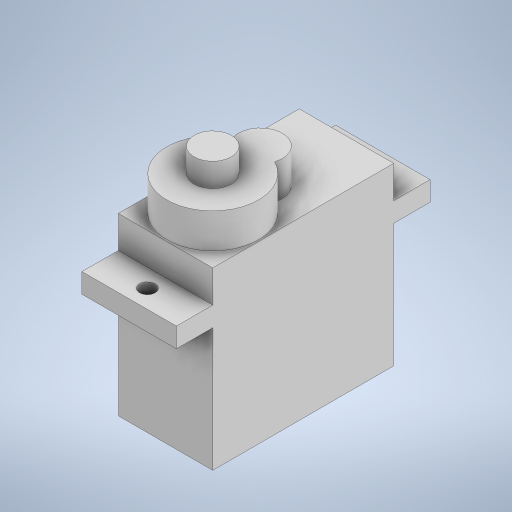
# Autodesk Inventor part: Servo Motor
Saved by Autodesk Inventor 2023 (Build 270158000, 158)
## iProperties
Created: 2023-03-09
Part Number: Servo Motor
Material: Generic
Document SubType Name: Modeling
Designer: 1roweste
Density: 1 g/cm^3
Appearance: Default
Author: 1roweste
Autodesk Inventor part; units mm, degrees
ref_plane "YZ Plane" through (0, 0, 0) normal (1, 0, 0) x (0, 1, 0)
sketch "Sketch1" plane through (0, 0, 0) normal (0, 1, 0) x (-1, 0, 0)
  line L0 (-6, 11.5) -> (6, 11.5)
  line L1 (6, 11.5) -> (6, -11.5)
  line L2 (6, -11.5) -> (-6, -11.5)
  line L3 (-6, -11.5) -> (-6, 11.5)
  point P0 (0, 0)
  point P1 (6, 0)
  point P2 (0, -11.5)
  dimension "d0" = 12
  dimension "d1" = 23
  dimension "d2" = 0
  dimension "d3" = 0
  constraints: 8 end point, 2 midpoint, 2 parallel, 1 horizontal, 1 perpendicular
  measures "d0" distance of L1.end L2.end
  measures "d1" distance of L0.end L1.end
  measures "d2" vertical distance of point (0, 0) point (6, 0)
  measures "d3" horizontal distance of point (0, 0) point (0, -11.5)
extrude "Extrusion1" add sketch "Sketch1" along normal blind 22.3
ref_plane "Work Plane1" through (0, 18.2, 0) normal (0, -1, 0) x (1, 0, 0)
sketch "Sketch2" plane through (0, 18.2, 0) normal (0, -1, 0) x (1, 0, 0)
  line L0 (-6, -11.5) -> (-6, 11.5) projected
  line L1 (-6, 11.5) -> (6, 11.5)
  line L2 (6, 11.5) -> (6, 16.125)
  line L3 (6, 16.125) -> (-6, 16.125)
  line L4 (-6, 16.125) -> (-6, 11.5)
  circle A0 centre (0, 13.8125) radius 1
  point P0 (0, 0)
  point P1 (0, 16.125)
  point P2 (6, 13.8125)
  dimension "d7" = 12
  dimension "d8" = 4.625
  dimension "d9" = 2
  dimension "d10" = 0
  dimension "d11" = 0
  constraints: 8 end point, 2 midpoint, 2 parallel, 1 centre point, 1 horizontal, 1 perpendicular
  measures "d7" distance of L3.end L2.end
  measures "d8" distance of L2.end L1.end
  measures "d9" diameter of A0
  measures "d10" horizontal distance of point (0, 16.125) A0.centre
  measures "d11" vertical distance of point (6, 13.812) A0.centre
extrude "Extrusion2" add sketch "Sketch2" along normal blind 2.5
ref_plane "Work Plane2" through (-6, 0, 0) normal (0, 0, 1) x (1, 0, 0)
mirror "Mirror1" about plane through (-6, 0, 0) normal (0, 0, 1) of "Extrusion2"
sketch "Sketch3" plane through (0, 22.3, 0) normal (0, 1, 0) x (1, 0, 0)
  line L0 (6, 11.5) -> (-6, 11.5) projected
  line L1 (-6, 11.5) -> (-6, -11.5) projected
  line L2 (-6, -11.5) -> (6, -11.5) projected
  line L3 (6, -11.5) -> (6, 11.5) projected
  circle A0 centre (0, -5.5) radius 5.85
  circle A1 centre (0, 0.55) radius 2.8
  point P0 (0, 0)
  point P1 (0, -11.5)
  point P2 (2.6696, -0.2946)
  point P3 (-2.6696, -0.2946)
  dimension "d16" = 11.7
  dimension "d17" = 0
  dimension "d18" = 6
  dimension "d21" = 5.6
  dimension "d22" = 0
  dimension "d23" = 6.05
  constraints: 2 centre point, 1 midpoint
  measures "d16" diameter of A0
  measures "d17" horizontal distance of A0.centre point (0, -11.5)
  measures "d18" distance from line of L2 A0.centre
  measures "d21" diameter of A1
  measures "d22" horizontal distance of A0.centre A1.centre
  measures "d23" distance of A0.centre A1.centre
extrude "Extrusion3" add sketch "Sketch3" along normal blind 4.4 contours A0 A1 | A1 A0 | A0 A1
sketch "Sketch4" plane through (0, 26.7, 0) normal (0, 1, 0) x (1, 0, 0)
  arc A0 (-2.6696, -0.2946) -> (2.6696, -0.2946) centre (0, -5.5) ccw projected
  arc A1 (2.6696, -0.2946) -> (-2.6696, -0.2946) centre (0, 0.55) ccw projected
  circle A2 centre (0, -5.5) radius 2.375
  point P0 (0, 0)
  dimension "d24" = 4.75
  constraints: 1 centre point, 1 coincident
  measures "d24" diameter of A2
extrude "Extrusion4" add sketch "Sketch4" along normal blind 3 contours A2
body "Solid1"
